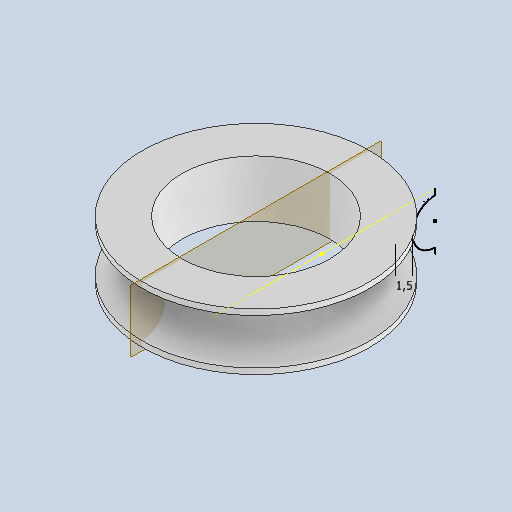
# Autodesk Inventor part: Umlenkfläche
Saved by Autodesk Inventor 2025 (Build 290162010, 162A)
## iProperties
Created: 2024-11-18
Part Number: Umlenkfläche
Material: PC/ABS-Kunststoff, Umlenkrolle
Document SubType Name: Modeling
Designer: Admin
Density: 1.1 g/cm^3
Appearance: Glatt - Weiß(1)
Mass: 0.600447 g
Surface Area: 9.74408 cm^2
Volume: 0.545861 cm^3
Author: Admin
Autodesk Inventor part; units mm, degrees
ref_plane "YZ Plane" through (0, 0, 0) normal (1, 0, 0) x (0, 1, 0)
ref_plane "XZ Plane" through (0, 0, 0) normal (0, 1, 0) x (-1, 0, 0)
ref_plane "XY Plane" through (0, 0, 0) normal (0, 0, 1) x (1, 0, 0)
sketch "Skizze1" plane through (0, 0, 0) normal (0, 0, 1) x (1, 0, 0)
  circle A0 centre (-5.7665, 0) radius 6.5 projected
  circle A1 centre (-5.7665, 0) radius 10
  point P0 (0, 0)
  dimension "d0" = 20
  constraints: 1 centre point, 1 coincident
  measures "d0" diameter of A1
sketch "Skizze2" plane through (0, 0, 0) normal (1, 0, 0) x (0, 1, 0)
  line L0 (6.5, 0) -> (-6.5, 0) construction
  line L1 (10, 0) -> (-10, 0) construction
  line L2 (10, 0) -> (10, -0.5)
  arc A0 (10, -0.5) -> (8, -2.5) centre (10, -2.5) ccw
  line L3 (6.5, -4.8) -> (6.5, -0.2) construction
  line L4 (8, -2.5) -> (6.5, -2.5) construction
  line L5 (10, -5) -> (10, -4.5)
  arc A1 (8, -2.5) -> (10, -4.5) centre (10, -2.5) ccw
  line L6 (8, -2.5) -> (8, -1.525) construction
  line L7 (10, -0.5) -> (8.7772, -0.5) construction
  point P0 (0, 0)
  dimension "d4" = 1.5
  constraints: 12 end point, 4 point on circle, 3 symmetric about line, 3 vertical, 2 centre point, 2 tangent, 1 horizontal, 1 midpoint, 1 perpendicular, 3 other
  measures "d4" distance of L4.start L4.end
ref_plane "Arbeitsebene1" through (-5.7665, 0, 0) normal (1, 0, 0) x (0, 1, 0)
sketch "Skizze3" plane through (-5.7665, 0, 0) normal (1, 0, 0) x (0, 1, 0)
  line L0 (10, 0) -> (10, -0.5) projected
  arc A0 (10, -0.5) -> (8, -2.5) centre (10, -2.5) ccw projected
  arc A1 (8, -2.5) -> (10, -4.5) centre (10, -2.5) ccw projected
  line L1 (10, -5) -> (10, -4.5) projected
  line L2 (10, -5) -> (6.5, -5)
  line L3 (6.5, -5) -> (6.5, 0)
  line L4 (6.5, 0) -> (10, 0)
  line L5 (6.5, -4.8) -> (6.5, -0.2)
  line L6 (6.3, -5) -> (-6.3, -5) projected
  point P0 (0, 0)
  dimension "d9" = 8
  constraints: 8 end point, 2 collinear, 2 perpendicular, 1 horizontal, 1 vertical, 2 other
  measures "d9" horizontal distance of point (0, 0) A0.end
sweep "Sweeping2" add profiles "Skizze3" path "Skizze1" path curves A1
